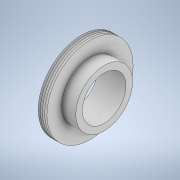
# Autodesk Inventor part: 轴套1
Saved by Autodesk Inventor 2020 (Build 240168000, 168)
## iProperties
Created: 2021-06-17
Part Number: 轴套1
Material: 常规
Document SubType Name: Modeling
Designer: dell
Density: 1 g/cm^3
Appearance: 默认
Author: dell
Autodesk Inventor part; units mm, degrees
ref_plane "YZ Plane" through (0, 0, 0) normal (1, 0, 0) x (0, 1, 0)
ref_plane "XZ Plane" through (0, 0, 0) normal (0, 1, 0) x (-1, 0, 0)
ref_plane "XY Plane" through (0, 0, 0) normal (0, 0, 1) x (1, 0, 0)
sketch "草图1" plane through (0, 0, 0) normal (0, 0, 1) x (1, 0, 0)
  line L0 (-31.2, 0) -> (5.2, 0) construction
  line L1 (0, -36.4) -> (0, 36.4) construction
  line L2 (-26, 22.5) -> (-13, 22.5)
  line L3 (-13, -22.5) -> (-26, -22.5)
  line L4 (-26, -22.5) -> (-26, 22.5)
  line L5 (-13, 26) -> (0, 26)
  line L6 (0, 26) -> (0, -26)
  line L7 (0, -26) -> (-13, -26)
  line L8 (-13, -26) -> (-13, -22.5)
  line L9 (-13, 22.5) -> (-13, 26)
  line L10 (-26, 20) -> (0, 20)
  line L11 (0, 20) -> (0, -20)
  line L12 (0, -20) -> (-26, -20)
  line L13 (-26, -20) -> (-26, 20)
  point P0 (0, 0)
  point P1 (0, 20)
  dimension "d0" = 26
  dimension "d1" = 13
  dimension "d2" = 45
  dimension "d3" = 52
  dimension "d4" = 40
  constraints: 24 end point, 6 parallel, 3 horizontal, 2 perpendicular, 2 point on line, 1 collinear, 1 midpoint, 3 other
  measures "d0" distance between parallel lines of L1 L4
  measures "d1" distance of L5.start L5.end
  measures "d2" distance between parallel lines of L3 L2
  measures "d3" distance between parallel lines of L7 L5
  measures "d4" distance between parallel lines of L12 L10
revolve "旋转1" add sketch "草图1" angle 360 about axis through (-10, 0, 0) along (1, 0, 0) contours L2 L9 L5 L6 L10 L4
sketch "草图2" plane through (0, 0, 0) normal (0, 0, 1) x (1, 0, 0)
  line L0 (-26, -22.5) -> (-26, 22.5) construction
  line L1 (-13, -22.5) -> (-13, 22.5) construction
  line L2 (-26, 22.5) -> (-13, 22.5) construction
  line L3 (-26, -22.5) -> (-13, -22.5) construction
  line L4 (-21, 39.5) -> (-13, 39.5)
  line L5 (-13, 39.5) -> (-13, -39.5)
  line L6 (-13, -39.5) -> (-21, -39.5)
  line L7 (-21, -39.5) -> (-21, 39.5)
  line L8 (-81.7478, 0) -> (13.6246, 0) construction
  line L9 (-21, 22.5) -> (-13, 22.5)
  line L10 (-21, 39.5) -> (-20, 37.7679)
  line L11 (-20, 37.7679) -> (-19, 39.5)
  line L12 (-19, 39.5) -> (-18, 37.7679)
  line L13 (-18, 37.7679) -> (-17, 39.5)
  line L14 (-17, 39.5) -> (-16, 37.7679)
  line L15 (-16, 37.7679) -> (-15, 39.5)
  line L16 (-15, 39.5) -> (-14, 37.7679)
  line L17 (-14, 37.7679) -> (-13, 39.5)
  point P0 (0, 0)
  dimension "d6" = 8
  dimension "d7" = 79
  dimension "d8" = 60
  dimension "d9" = 2
  dimension "d10" = 2
  constraints: 26 end point, 7 equal length, 4 point on line, 3 parallel, 2 collinear, 1 horizontal, 1 midpoint, 1 perpendicular, 1 other
  measures "d6" distance between parallel lines of L5 L7
  measures "d7" distance between parallel lines of L6 L4
  measures "d8" angle of L4 L10
  measures "d9" distance of L4.start L11.end
  measures "d10" distance of L13.end L11.end
revolve "旋转2" add sketch "草图2" angle 360 about axis through (-10, 0, 0) along (1, 0, 0) contours L10 L11 L12 L13 L14 L15 L16 L17 L5 L9 L7
